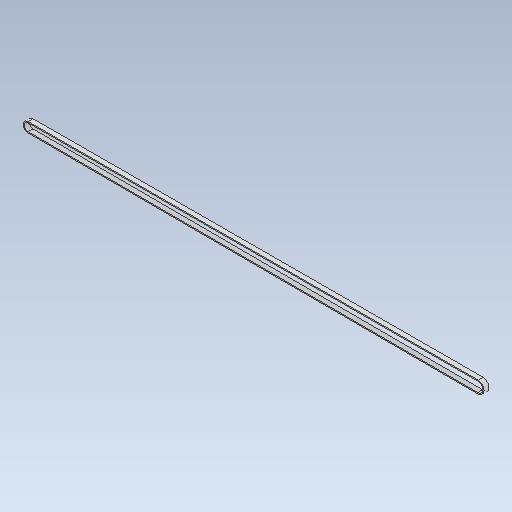
# Autodesk Inventor part: z-belt
Saved by Autodesk Inventor 2020.4 (Build 244396000, 396)
## iProperties
Created: 2021-03-30
Part Number: z-belt
Material: Generic
Document SubType Name: Modeling
Designer: AOB
Density: 1 g/cm^3
Appearance: Default
Mass: 9.13606 g
Surface Area: 167.034 cm^2
Volume: 9.13606 cm^3
Author: AOB
Autodesk Inventor part; units mm, degrees
ref_plane "YZ Plane" through (0, 0, 0) normal (1, 0, 0) x (0, 1, 0)
ref_plane "XZ Plane" through (0, 0, 0) normal (0, 1, 0) x (-1, 0, 0)
ref_plane "XY Plane" through (0, 0, 0) normal (0, 0, 1) x (1, 0, 0)
sketch "Sketch1" plane through (0, 0, 0) normal (0, 0, 1) x (1, 0, 0)
  arc A0 (0, 4.7) -> (0, -4.7) centre (0, 0) ccw
  arc A1 (549.5802, -6.0956) -> (549.5802, 6.0956) centre (550, 0) ccw
  line L0 (0, 4.7) -> (550.3888, 6.0976)
  line L1 (550.3888, -6.0976) -> (0, -4.7)
  line L2 (550.4201, 6.0955) -> (550.4201, 7.4355) construction
  line L3 (0, 4.7) -> (0, 6.0378) construction
  arc A2 (0, 6.0378) -> (-0.0153, -6.0378) centre (0, 0) ccw
  arc A3 (550.4198, -7.4356) -> (550.4201, 7.4355) centre (550, 0) ccw
  line L4 (0, 6.0378) -> (550.4201, 7.4355)
  line L5 (550.4198, -7.4356) -> (-0.0153, -6.0378)
  dimension "d0" = 9.4
  dimension "d1" = 12.22
  dimension "d6" = 550
  constraints: 12 end point, 11 point on circle, 4 centre point, 3 coincident, 2 parallel, 2 point on line, 2 vertical, 1 tangent
  measures "d0" diameter of A0
  measures "d1" diameter of A1
  measures "d6" distance of A1.centre point (0, 0)
extrude "Extrusion1" add sketch "Sketch1" along normal blind 6
body "Solid1"
